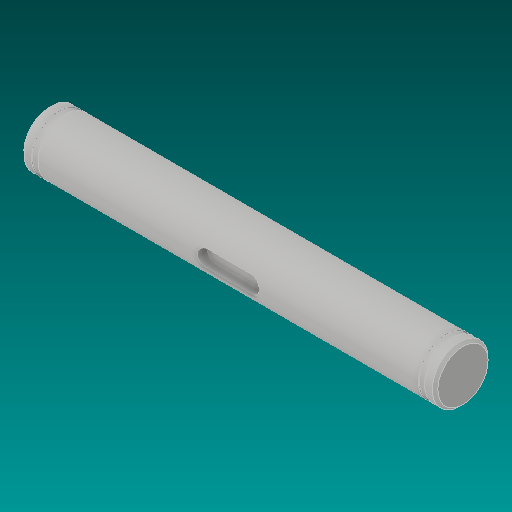
# Autodesk Inventor part: NSFMRRA10-74-B3-S3-KC31.5-A11(000_000)_s
Saved by Autodesk Inventor 2020 (Build 240168000, 168)
## iProperties
Created: 2022-11-16
Part Number: NSFMRRA10-74-B3-S3-KC31.5-A11(000_000)_s
Material: Generic
Catalog Web Link: www.cadenas.de
Description: NSFMRR, SFMRR, PSFMRR, SSFMRR, NSFHRR, SFHRR, PSFHRR, SSFHRR, NSFRR, SFRR, PSFRR, SSFRR, NSFMRRA, SFMRRA, PSFMRRA, SSFMRRA, NSFHRRA, SFHRRA, PSFHRRA, SSFHRRA, NSFRRA, SFRRA, PSFRRA, SSFRRA, HFRRA, PHFRRA, PSFRR PSFRRA, PSFHRR, PSFHRRA, SSFRR, SSFRRA, SSFHRR, SSFHRRA, PPSFRR, PPSFRRA, PPSFHRR, PPSFHRRA, SSSFRR, SSSFRRA, SSSFHRR, SSSFHRRA_shaft-Rotary Shafts - Retaining Ring Grooves on Both Ends - Standard
Vendor: MISUMI
Document SubType Name: Modeling
Designer: psAdmin
Manufacturer: MISUMI
Mass: 5.73651 g
Surface Area: 25.2511 cm^2
Volume: 5.73651 cm^3
Density: 1 g/cm^3
Appearance: PSOLRGB-175-175-175
Category: PARTsolutions
Company: MISUMI
PSOL_IDENT_0: {$CADENAS_DATA/23d-libs/misumi/metric/11_rotary_shafts/11_components/psfrra/psfrra.prj},808 {VTYP=3D
PSOL_IDENT_1: },{NB=NSFMRRA10-74-B3-S3-KC31.5-A11(000_000)_s},{LINA=NSFMRRA10-74-B3-S3-KC31.5-A11},{NN=NSFMRR, SFM
PSOL_IDENT_2: RR, PSFMRR, SSFMRR, NSFHRR, SFHRR, PSFHRR, SSFHRR, NSFRR, SFRR, PSFRR, SSFRR, NSFMRRA, SFMRRA, PSFMR
PSOL_IDENT_3: RA, SSFMRRA, NSFHRRA, SFHRRA, PSFHRRA, SSFHRRA, NSFRRA, SFRRA, PSFRRA, SSFRRA, HFRRA, PHFRRA, PSFRR
PSOL_IDENT_4: PSFRRA, PSFHRR, PSFHRRA, SSFRR, SSFRRA, SSFHRR, SSFHRRA, PPSFRR, PPSFRRA, PPSFHRR, PPSFHRRA, SSSFRR,
PSOL_IDENT_5: SSSFRRA, SSSFHRR, SSSFHRRA_shaft},{DATE=21.04.2022 07:40:13},{GEOMDATE=27.07.2021 07:13:06},{VERSIO
PSOL_IDENT_6: N=},{LINEID=30},{WBVAR=TS,TYS,MAT,ST,ALT1,L,B,S,ALT2,KC,A,WKC,C,K,E,KZ,Z,ALT3,FC,GALT3,WFC,J,WALT3,V
PSOL_IDENT_7: ,ALT4,SFC,SG,AG,ALT5,UC,ALT7,SC,ALT10,KWC,ALT11,WC,ALT32,CD,ALT34,TCJ,WTCJ,XT,HCJ,WHCJ,XH},{WBNUMERI
PSOL_IDENT_8: C=L,B,S,KC,A,WKC,C,K,E,KZ,Z,FC,GALT3,WFC,J,WALT3,V,SFC,SG,AG,UC,SC,KWC,WC,TCJ,WTCJ,XT,HCJ,WHCJ,XH}
PSOL_IDENT_9: {NB=NSFMRRA10-74-B3-S3-KC31.5-A11(000_000)_s},{LINA=NSFMRRA10-74-B3-S3-KC31.5-A11},{KT=DUMMY},{PN=NS
PSOL_IDENT_10: FMRRA10-74-B3-S3-KC31.5-A11},{TYPE=NSFMRRA},{TS=SWR},{TYS=H9},{TYSALG= 'H9','h9 (Cold-drawn)','H7','
PSOL_IDENT_11: h7 (Ground)','G6','g6 (Ground)' },{MAT=S45C},{MATALG= 'S45C','S45C Equivalent', 'SUS304','SUS304' },
PSOL_IDENT_12: {ST=},{STALG= '','' },{D=10.0},{ALT1=},{ALT1ALG= '','w/o LKC (Changes L Tolerance)','-LKC','with LKC
PSOL_IDENT_13: (Changes L Tolerance)' },{L=74.0},{LALG=[15:800/0.1]},{LMIN=15},{LMAX=800},{NOTE=25},{B=3.0},{BALG=
PSOL_IDENT_14: [3:70/0.1]},{BMAX=70},{S=3.0},{SALG=[3:69/0.1]},{SMAX=69},{MM=1.15},{DD=9.6},{ARR=STWS10},{ALT2=KC},
PSOL_IDENT_15: {ALT2ALG= '', 'w/o Key Grooves','KC','with KC (Key Groove)','WKC','with WKC (Two Key Grooves)','KCWK
PSOL_IDENT_16: C','with KC + WKC (Three Key Grooves)','KZ','with KC + WKC + KZ (Four Key Grooves)' },{ALT2PN=-KC31.
PSOL_IDENT_17: 5-A11},{KC=31.5},{KCALG=[0:71/0.1]},{KCMIN=0},{KCMAX=71},{A=11.0},{AALG=[3:42.5/0.1]},{AMIN=3},{AMAX=
PSOL_IDENT_18: 42.5},{WKC=0.0},{WKCALG=[0]},{WKCMIN=0},{WKCMAX=0},{C=0.0},{CALG=[0]},{CMIN=3},{CMAX=0},{K=0.0},{KAL
PSOL_IDENT_19: G=[0]},{KMIN=0},{KMAX=69},{E=0.0},{EALG=[0]},{EMIN=3},{EMAX=72},{KZ=0.0},{KZALG=[0]},{KZMIN=76},{KZM
PSOL_IDENT_20: AX=71},{Z=0.0},{ZALG=[0]},{ZMIN=3},{ZMAX=74},{CIFKC=2},{CIFWKC=1},{CIFK=1},{CIFKZ=2},{PCUT3D=0},{QCU
PSOL_IDENT_21: T3D=0},{BB=3},{BBALT2=3},{TT=1.8},{TTALT2=1.8},{ALT3=},{ALT3ALG= '', 'w/o Set Screw Flat','FC','with
PSOL_IDENT_22: FC (Adds a Set Screw Flat)','WFC','with WFC (Adds Two Set Screw Flats)','FCWFC','with FC + WFC (Add
PSOL_IDENT_23: s Three Set Screw Flats)' },{ALT3PN=},{FC=0},{FCALG=[0]},{FCMIN=0},{FCMAX=73},{GALT3=0},{GALT3ALG=[0
PSOL_IDENT_24: ]},{GALT3MIN=1},{GALT3MAX=70},{GALT3MAX2=68},{GALT3MAX3=70},{WFC=0},{WFCALG=[0]},{WFCMIN=0},{WFCMIN2=
PSOL_IDENT_25: 2},{WFCMAX=70},{WFCMAX2=-3},{WFCMAX3=-4},{J=0},{JALG=[0]},{JMIN=1},{JMAX=70},{JMAX2=-2},{JMAX3=-5},{
PSOL_IDENT_26: WALT3=0},{WALT3ALG=[0]},{WALT3MIN=0},{WALT3MIN2=76},{WALT3MAX=71},{WALT3MAX2=71},{V=0},{VALG=[0]},{V
PSOL_IDENT_27: MIN=1},{VMAX=70},{VMAX2=70},{CIFFC=0},{H=0},{ALT4=},{ALT4ALG= '', 'w/o SFC (2 Set Screw Flats (Angle
PSOL_IDENT_28: Specified))', 'SFC'  , 'with SFC (2 Set Screw Flats (Angle Specified))'},{ALT4PN=},{SFC=0},{SFCALG=
PSOL_IDENT_29: [0]},{SFCMIN=0},{SFCMAX=73},{SG=0},{SGALG=[0]},{SGMIN=1},{SGMAX=70},{AG=0},{AGALG=[0]},{CIFSFC=0},{A
PSOL_IDENT_30: LT5=},{ALT5ALG= '', 'w/o UC (Slit Cam Groove)', 'UC', 'with UC (Slit Cam Groove)'},{ALT5PN=},{UC=0},
PSOL_IDENT_31: {UCALG=[0]},{UCMIN=1},{UCMAX=68},{DDALT5=8},{LL1=0},{ALT7=},{ALT7ALG= '', 'w/o SC (Wrench Flats)', '
PSOL_IDENT_32: SC', 'with SC (Wrench Flats)'},{ALT7PN=},{SC=0},{SCALG=[0]},{SCMIN=0},{SCMAX=74},{WALT7=0},{LL2=0},{
PSOL_IDENT_33: CIFSC=0},{ALT10=},{ALT10ALG= '','Not applicable' },{ALT10PN=},{KWC=0},{KWCALG=[0]},{KWCMIN=1},{KWCMA
PSOL_IDENT_34: X=0},{WALT10=8},{ALT11=},{ALT11ALG= '','Not applicable' },{ALT11PN=},{WC=0.0},{WCALG=[0]},{ALT32=},{
PSOL_IDENT_35: ALT32ALG=  '','w/o CD (Changes Part D Chamfering)','-CD', 'with CD (Changes Part D Chamfering)' },{C
PSOL_IDENT_36: D=},{CDALG= '','N/A' },{CD3D=0.5},{CIF32=0},{CIF320=0},{CIF32B=0},{CIF32S=0},{ALT32PN=},{ERRORPN=},{
PSOL_IDENT_37: ERRORRALT2=OK},{ERRORRALT3=OK},{ERRORRALT4=NG},{ERRORRALT5=NG},{ERRORRALT7=NG},{ERRORRALT10=OK},{ERR
PSOL_IDENT_38: ORALT23=OK},{ERRORALT24=OK},{ERRORALT25=OK},{ERRORALT27=OK},{ERRORALT210=OK},{ERRORALT34=OK},{ERRORA
PSOL_IDENT_39: LT35=OK},{ERRORALT37=OK},{ERRORALT310=OK},{ERRORALT45=OK},{ERRORALT47=OK},{ERRORALT410=OK},{ERRORALT
PSOL_IDENT_40: 75=OK},{ERRORALT510=OK},{ERRORALT710=OK},{ALT34=},{ALT34ALG= '','Not applicable'},{TCJ=0},{WTCJ=0},{
PSOL_IDENT_41: XT=0},{TM=4},{TCJALG=[0]},{TCJMIN=7.000},{TCJMAX=34.000},{TCJMAX1=34.000},{HCJ=0},{WHCJ=0},{XH=0},{H
PSOL_IDENT_42: P=4},{HCJALG=[0]},{HCJMIN=7.000},{HCJMAX=34.000},{HCJMAX1=34.000},{LCJ=0},{LMINX=15},{XALG=[0]},{XCJ
PSOL_IDENT_43: MIN=7},{WTCJALG=[0]},{WHCJALG=[0]},{XHALG=[0]}
NB: NSFMRRA10-74-B3-S3-KC31.5-A11(000_000)_s
NN: NSFMRR, SFMRR, PSFMRR, SSFMRR, NSFHRR, SFHRR, PSFHRR, SSFHRR, NSFRR, SFRR, PSFRR, SSFRR, NSFMRRA, SFMRRA, PSFMRRA, SSFMRRA, NSFHRRA, SFHRRA, PSFHRRA, SSFHRRA, NSFRRA, SFRRA, PSFRRA, SSFRRA, HFRRA, PHFRRA, PSFRR PSFRRA, PSFHRR, PSFHRRA, SSFRR, SSFRRA, SSFHRR, SSFHRRA, PPSFRR, PPSFRRA, PPSFHRR, PPSFHRRA, SSSFRR, SSSFRRA, SSSFHRR, SSSFHRRA_shaft
NT: Rotary Shafts - Retaining Ring Grooves on Both Ends - Standard
NBSYN: $PN.($ALT34.$TCJ.$WTCJ.$XT._$HCJ.$WHCJ.$XH.)_s
LINA: NSFMRRA10-74-B3-S3-KC31.5-A11
CATALOG: Misumi
PN: NSFMRRA10-74-B3-S3-KC31.5-A11
TS: With Retaining Ring
TYS: h9 (Cold-drawn)
MAT: S45C Equivalent
D: 10
ALT1: w/o LKC (Changes L Tolerance)
L: 74
B: 3
S: 3
MM: 1.15
DD: 9.6
ALT2: with KC (Key Groove)
KC: 31.5
A: 11
WKC: 0
C: 0
K: 0
E: 0
KZ: 0
Z: 0
ALT3: w/o Set Screw Flat
FC: 0
GALT3: 0
WFC: 0
J: 0
WALT3: 0
V: 0
ALT4: w/o SFC (2 Set Screw Flats (Angle Specified))
SFC: 0
SG: 0
AG: 0
ALT5: w/o UC (Slit Cam Groove)
UC: 0
ALT7: w/o SC (Wrench Flats)
SC: 0
ALT10: Not applicable
KWC: 0
ALT11: Not applicable
WC: 0
ALT32: w/o CD (Changes Part D Chamfering)
CD: N/A
ALT34: Not applicable
TCJ: 0
WTCJ: 0
XT: 0
HCJ: 0
WHCJ: 0
XH: 0
SUPPLIER: MISUMI
ARTICLENO: NSFMRRA10-74-B3-S3-KC31.5-A11(000_000)_s
BOMINFO: NSFMRRA10-74-B3-S3-KC31.5-A11
CREATOR: CADENAS GmbH
d7: 0.000 mm
Title: NSFMRRA10-74-B3-S3-KC31.5-A11
Author: Cadenas PARTsolutions
Comments: Rotary Shafts - Retaining Ring Grooves on Both Ends - Standard
Autodesk Inventor part; units mm, degrees
ref_plane "YZ Plane" through (0, 0, 0) normal (1, 0, 0) x (0, 1, 0)
ref_plane "XZ Plane" through (0, 0, 0) normal (0, 1, 0) x (-1, 0, 0)
ref_plane "XY Plane" through (0, 0, 0) normal (0, 0, 1) x (1, 0, 0)
sketch "Sketch_1" plane through (0, 0, 0) normal (0, 0, 1) x (1, 0, 0)
  line L0 (74, 0) -> (0, 0)
  line L1 (0, 0) -> (0, 4.5)
  line L2 (0, 4.5) -> (0.5, 5)
  line L3 (0.5, 5) -> (73.5, 5)
  line L4 (73.5, 5) -> (74, 4.5)
  line L5 (74, 4.5) -> (74, 0)
  line L6 (74, 0) -> (0, 0)
  constraints: 14 end point
revolve "Revolution1" add sketch "Sketch_1" angle 360 about axis through (74, 0, 0) along (1, 0, 0)
sketch "_____10" plane through (0, 0, 5) normal (0, 0, 1) x (1, 0, 0)
  arc A0 (33, 1.5) -> (33, -1.5) centre (33, 0) ccw
  line L0 (33, -1.5) -> (41, -1.5)
  arc A1 (41, -1.5) -> (41, 1.5) centre (41, 0) ccw
  line L1 (41, 1.5) -> (33, 1.5)
  constraints: 4 end point, 4 point on circle, 2 centre point
extrude "Extrusion1" cut sketch "_____10" against normal blind 1.8
sketch "_____5" plane through (3, 0, 0) normal (1, 0, 0) x (0, 0, -1)
  circle A0 centre (0, 0) radius 10
  circle A1 centre (0, 0) radius 4.8
  constraints: 2 centre point
extrude "Extrusion2" cut sketch "_____5" against normal blind 1.15
sketch "_____6" plane through (71, 0, 0) normal (1, 0, 0) x (0, 0, -1)
  circle A0 centre (0, 0) radius 10
  circle A1 centre (0, 0) radius 4.8
  constraints: 2 centre point
extrude "Extrusion3" cut sketch "_____6" along normal blind 1.15
ref_plane "COMBINATION_MODULE_XY" through (0, 0, 0) normal (1, 0, 0) x (0, 0, -1)
ref_plane "COMBINATION_MODULE_YZ" through (0, 0, 0) normal (0, 0, -1) x (0, 1, 0)
ref_plane "COMBINATION_MODULE_ZX" through (0, 0, 0) normal (0, 1, 0) x (1, 0, 0)
ref_plane "to_ring_b_XY" through (2.425, 0, 0) normal (1, 0, 0) x (0, 0, -1)
ref_plane "to_ring_b_YZ" through (2.425, 0, 0) normal (0, 0, -1) x (0, 1, 0)
ref_plane "to_ring_b_ZX" through (2.425, 0, 0) normal (0, 1, 0) x (1, 0, 0)
ref_plane "to_ring_s_XY" through (71.575, 0, 0) normal (1, 0, 0) x (0, 0, -1)
ref_plane "to_ring_s_YZ" through (71.575, 0, 0) normal (0, 0, -1) x (0, 1, 0)
ref_plane "to_ring_s_ZX" through (71.575, 0, 0) normal (0, 1, 0) x (1, 0, 0)
body "Solid1"
